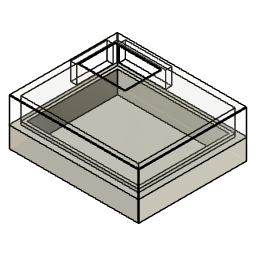
Case3D (Autodesk Fusion 360 design; units mm, degrees)
Autodesk Fusion 360 part; units mm, degrees
note: some values were not read from the file. Chosen so that the rebuilt part matches the saved one: which bodies a step acts on; which face or edge a step refers to.
sketch "Sketch2" plane through (0, 0, 1.57) normal (0, 0, 1) x (-1, 0, 0)
  line L0 (-160.46, -12.24) -> (-96.06, -12.24)
  line L1 (-96.06, -12.24) -> (-96.06, -66.17)
  line L2 (-96.06, -66.17) -> (-160.46, -66.17)
  line L3 (-160.46, -66.17) -> (-160.46, -12.24)
extrude "Extrude5" add sketch "Sketch2" along normal blind 20 makes body 1
sketch "Sketch3" plane through (0, 12.24, 0) normal (0, -1, 0) x (1, 0, 0)
  line L0 (96.06, 1.57) -> (160.46, 1.57)
  line L1 (160.46, 1.57) -> (160.46, 21.57)
  line L2 (160.46, 21.57) -> (96.06, 21.57)
  line L3 (96.06, 21.57) -> (96.06, 1.57)
  line L4 (79, 13.57) -> (170, 13.57)
  dimension "d13" = 8
  constraint perpendicular L1 L4
  measures "d13" distance of L2 L4
split "Split1" by curves path "Sketch3" along L4 bodies 1 makes body 2 at (138.9933, 30.2167, 1.57)
sketch "Sketch4" plane through (0, 0, 13.57) normal (0, 0, -1) x (1, 0, 0)
  line L0 (160.46, -66.17) -> (160.46, -12.24)
  line L1 (160.46, -12.24) -> (96.06, -12.24)
  line L2 (96.06, -12.24) -> (96.06, -66.17)
  line L3 (96.06, -66.17) -> (160.46, -66.17)
  line L4 (99.06, -63.17) -> (157.46, -63.17)
  line L5 (157.46, -63.17) -> (157.46, -15.24)
  line L6 (157.46, -15.24) -> (99.06, -15.24)
  line L7 (99.06, -15.24) -> (99.06, -63.17)
  line L8 (100.56, -61.67) -> (155.96, -61.67)
  line L9 (155.96, -61.67) -> (155.96, -16.74)
  line L10 (155.96, -16.74) -> (100.56, -16.74)
  line L11 (100.56, -16.74) -> (100.56, -61.67)
extrude "Extrude8" cut sketch "Sketch4" along normal blind 11 contours L8 L9 L10 L11 bodies 2
extrude "Extrude9" cut sketch "Sketch4" against normal blind 7 contours L8 L9 L10 L11 bodies 1
extrude "Extrude10" cut sketch "Sketch4" along normal blind 1.5 contours L0 L1 L2 L3 bodies 2
extrude "Extrude11" add sketch "Sketch4" along normal blind 1.5 contours L0 L1 L2 L3 bodies 1
move_body "Move1" bodies 1 2 to x (1, 0, 0) y (0, 1, 0) z (0, 0, 1) at (0, 0, -13)
move_body "Move2" bodies 2 to x (1, 0, 0) y (0, 1, 0) z (0, 0, 1) at (0, 0, -0.6)
extrude "Extrude12" add 1 faces at (138.9933, 30.2167, 8.57) along direction (0, 0, 1) blind 2 on bodies 1 bodies 1
extrude "Extrude13" cut 1 faces at (119.0267, 31.7167, 7.57) along direction (0, 0, 1) blind 2 on bodies 1 bodies 1
extrude "Extrude14" add 1 faces at (138.9933, 30.2167, 10.57) along direction (0, 0, 1) blind 2 on bodies 1 bodies 1
extrude "Extrude15" cut 1 faces at (119.0267, 31.7167, 9.57) along direction (0, 0, 1) blind 1 on bodies 1 bodies 1
extrude "Extrude16" cut 1 faces at (119.0267, 31.7167, 10.57) along direction (0, 0, 1) blind 0.5 on bodies 1 bodies 1
move_body "Move3" bodies 1 to x (1, 0, 0) y (0, 1, 0) z (0, 0, 1) at (0, 0, -0.6)
extrude "Extrude17" add 1 faces at (119.0267, 31.7167, 10.47) along direction (0, 0, -1) blind 11 on bodies 1 bodies 1
extrude "Extrude18" cut 1 faces at (119.0267, 31.7167, -0.53) along direction (0, 0, 1) blind 10 on bodies 1 bodies 1
extrude "Extrude19" cut 1 faces at (137.4933, 15.74, -0.03) along direction (0, 0, 1) blind 10 on bodies 1 bodies 1
extrude "Extrude20" cut 1 faces at (119.0267, 31.7167, 9.47) along direction (0, 0, 1) blind 0.5 on bodies 1 bodies 1
sketch "Sketch5" plane through (0, 0, 11.97) normal (0, 0, 1) x (-1, 0, 0)
  line L0 (-160.46, -66.17) -> (-96.06, -66.17)
  line L1 (-96.06, -66.17) -> (-96.06, -12.24)
  line L2 (-96.06, -12.24) -> (-160.46, -12.24)
  line L3 (-160.46, -12.24) -> (-160.46, -66.17)
  line L4 (-100, -43) -> (-123, -43)
  line L5 (-123, -43) -> (-123, -61)
  line L6 (-123, -61) -> (-100, -61)
  line L7 (-100, -61) -> (-100, -43)
  constraint horizontal L4
  constraint vertical L5
  constraint horizontal L6
  constraint vertical L7
extrude "Extrude21" cut sketch "Sketch5" against normal blind 5 contours L4 L5 L6 L7 bodies 1
extrude "Extrude22" add 1 faces at (147.9733, 40.47, 11.97) along direction (0, 0, 1) blind 1 on bodies 1 bodies 1
extrude "Extrude23" cut 1 faces at (145.9733, 40.47, 9.97) along direction (0, 0, 1) blind 1 on bodies 1 bodies 1
extrude "Extrude24" cut 1 faces at (145.9733, 40.47, 10.97) along direction (0, 0, 1) blind 1 on bodies 1 bodies 1
extrude "Extrude25" add 1 faces at (145.9733, 40.47, 11.97) along direction (0, 0, -1) blind 1 on bodies 1 bodies 1
extrude "Extrude26" cut 1 faces at (147.9733, 40.47, 12.97) along direction (0, 0, -1) blind 1.5 on bodies 1 bodies 1
sketch "Sketch7" plane through (96.06, 0, 0) normal (-1, 0, 0) x (0, -1, 0)
  line L0 (-12.24, 11.47) -> (-66.17, 11.47)
  line L1 (-66.17, 11.47) -> (-66.17, -1.53)
  line L2 (-66.17, -1.53) -> (-12.24, -1.53)
  line L3 (-12.24, -1.53) -> (-12.24, 11.47)
  line L4 (-61, 10.5) -> (-42.9738, 10.5)
  line L5 (-42.9738, 10.5) -> (-42.9738, 1.6958)
  line L6 (-42.9738, 1.6958) -> (-61, 1.6958)
  line L7 (-61, 1.6958) -> (-61, 10.5)
  constraint horizontal L4
  constraint vertical L5
  constraint horizontal L6
  constraint vertical L7
extrude "Extrude27" cut sketch "Sketch7" against normal blind 5 contours L4 L5 L6 L7 bodies 1
sketch "Sketch8" plane through (0, 66.17, 0) normal (0, 1, 0) x (-1, 0, 0)
  line L0 (-96.06, 11.47) -> (-160.46, 11.47)
  line L1 (-160.46, 11.47) -> (-160.46, -1.53)
  line L2 (-160.46, -1.53) -> (-96.06, -1.53)
  line L3 (-96.06, -1.53) -> (-96.06, 11.47)
  line L4 (-123, 10) -> (-100.0139, 10)
  line L5 (-100.0139, 10) -> (-100.0139, 1.7153)
  line L6 (-100.0139, 1.7153) -> (-123, 1.7153)
  line L7 (-123, 1.7153) -> (-123, 10)
  constraint horizontal L4
  constraint vertical L5
  constraint horizontal L6
  constraint vertical L7
extrude "Extrude28" cut sketch "Sketch8" against normal blind 4 contours L4 L5 L6 L7 bodies 1
fillet "Fillet1" radius 0.3 4 edges at (96.06, 39.205, 11.47) (128.26, 66.17, 11.47) (160.46, 39.205, 11.47) (128.26, 12.24, 11.47) on bodies 1
fillet "Fillet2" radius 0.3 16 edges at (96.1479, 66.0821, 11.3821) (96.06, 66.17, 4.82) (96.06, 12.24, 4.82) (96.1479, 12.3279, 11.3821) (160.3721, 66.0821, 11.3821) (160.46, 66.17, 4.82) (160.3721, 12.3279, 11.3821) (160.46, 12.24, 4.82) (96.06, 66.17, -6.78) (96.06, 12.24, -6.78) (96.06, 39.205, -12.03) (128.26, 66.17, -12.03) (160.46, 66.17, -6.78) (160.46, 39.205, -12.03) (160.46, 12.24, -6.78) (128.26, 12.24, -12.03) on bodies 1 2
named bodies: "TampaSuperior", "TampaInferior"
